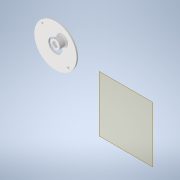
# Autodesk Inventor part: Anglerfish_Lightplate_Tosslink
Saved by Autodesk Inventor 2022 (Build 260153000, 153)
## iProperties
Created: 2022-07-21
Part Number: Anglerfish_Lightplate_Tosslink
Material: Generisch
Document SubType Name: Modeling
Designer: Muriel
Density: 1 g/cm^3
Appearance: Vorgabe
Author: Muriel
Autodesk Inventor part; units mm, degrees
ref_plane "YZ Plane" through (0, 0, 0) normal (1, 0, 0) x (0, 1, 0)
ref_plane "XZ Plane" through (0, 0, 0) normal (0, 1, 0) x (-1, 0, 0)
ref_plane "XY Plane" through (0, 0, 0) normal (0, 0, 1) x (1, 0, 0)
ref_plane "Arbeitsebene1" through (98.0402, -40.0393, 0) normal (0, 0, 1) x (1, 0, 0)
sketch "Skizze1" plane through (98.0402, -40.0393, 0) normal (0, 0, 1) x (1, 0, 0)
  arc A0 (-132.5402, 32.1532) -> (-131.9673, 30.3899) centre (-129.5402, 32.1532) ccw projected
  line L0 (-119.9354, 13.8294) -> (-131.9673, 30.3899) projected
  arc A1 (-119.9354, 13.8294) -> (-118.4354, 12.7395) centre (-117.5083, 15.5927) ccw projected
  line L1 (-98.9673, 6.414) -> (-118.4354, 12.7395) projected
  arc A2 (-98.9673, 6.414) -> (-97.1132, 6.414) centre (-98.0402, 9.2672) ccw projected
  line L2 (-77.6451, 12.7395) -> (-97.1132, 6.414) projected
  arc A3 (-77.6451, 12.7395) -> (-76.1451, 13.8294) centre (-78.5722, 15.5927) ccw projected
  line L3 (-64.1132, 30.3899) -> (-76.1451, 13.8294) projected
  arc A4 (-64.1132, 30.3899) -> (-63.5402, 32.1532) centre (-66.5402, 32.1532) ccw projected
  line L4 (-63.5402, 52.6232) -> (-63.5402, 32.1532) projected
  arc A5 (-63.5402, 52.6232) -> (-64.1132, 54.3865) centre (-66.5402, 52.6232) ccw projected
  line L5 (-76.1451, 70.9471) -> (-64.1132, 54.3865) projected
  arc A6 (-76.1451, 70.9471) -> (-77.6451, 72.0369) centre (-78.5722, 69.1837) ccw projected
  line L6 (-97.1132, 78.3624) -> (-77.6451, 72.0369) projected
  arc A7 (-97.1132, 78.3624) -> (-98.9673, 78.3624) centre (-98.0402, 75.5093) ccw projected
  line L7 (-118.4354, 72.0369) -> (-98.9673, 78.3624) projected
  arc A8 (-118.4354, 72.0369) -> (-119.9354, 70.9471) centre (-117.5083, 69.1837) ccw projected
  line L8 (-131.9673, 54.3865) -> (-119.9354, 70.9471) projected
  arc A9 (-131.9673, 54.3865) -> (-132.5402, 52.6232) centre (-129.5402, 52.6232) ccw projected
  line L9 (-132.5402, 32.1532) -> (-132.5402, 52.6232) projected
  circle A10 centre (-98.0403, 42.3882) radius 10
  arc A11 (-132.5402, 32.1532) -> (-131.9673, 30.3899) centre (-129.5402, 32.1532) ccw projected
  line L10 (-119.9354, 13.8294) -> (-131.9673, 30.3899) projected
  arc A12 (-119.9354, 13.8294) -> (-118.4354, 12.7395) centre (-117.5083, 15.5927) ccw projected
  line L11 (-98.9673, 6.414) -> (-118.4354, 12.7395) projected
  arc A13 (-98.9673, 6.414) -> (-97.1132, 6.414) centre (-98.0402, 9.2672) ccw projected
  line L12 (-77.6451, 12.7395) -> (-97.1132, 6.414) projected
  arc A14 (-77.6451, 12.7395) -> (-76.1451, 13.8294) centre (-78.5722, 15.5927) ccw projected
  line L13 (-64.1132, 30.3899) -> (-76.1451, 13.8294) projected
  arc A15 (-64.1132, 30.3899) -> (-63.5402, 32.1532) centre (-66.5402, 32.1532) ccw projected
  line L14 (-63.5402, 52.6232) -> (-63.5402, 32.1532) projected
  arc A16 (-63.5402, 52.6232) -> (-64.1132, 54.3865) centre (-66.5402, 52.6232) ccw projected
  line L15 (-76.1451, 70.9471) -> (-64.1132, 54.3865) projected
  arc A17 (-76.1451, 70.9471) -> (-77.6451, 72.0369) centre (-78.5722, 69.1837) ccw projected
  line L16 (-97.1132, 78.3624) -> (-77.6451, 72.0369) projected
  arc A18 (-97.1132, 78.3624) -> (-98.9673, 78.3624) centre (-98.0402, 75.5093) ccw projected
  line L17 (-118.4354, 72.0369) -> (-98.9673, 78.3624) projected
  arc A19 (-118.4354, 72.0369) -> (-119.9354, 70.9471) centre (-117.5083, 69.1837) ccw projected
  line L18 (-131.9673, 54.3865) -> (-119.9354, 70.9471) projected
  arc A20 (-131.9673, 54.3865) -> (-132.5402, 52.6232) centre (-129.5402, 52.6232) ccw projected
  line L19 (-132.5402, 32.1532) -> (-132.5402, 52.6232) projected
  circle A21 centre (-88.5403, 53.3903) radius 1.352 projected
  circle A22 centre (-98.0403, 42.3903) radius 3.6574 projected
  circle A23 centre (-98.0403, 42.3903) radius 30
  dimension "d0" = 20
  dimension "d21" = 60
  constraints: 2 centre point, 2 coincident
  measures "d0" diameter of A10
  measures "d21" diameter of A23
extrude "Extrusion1" add sketch "Skizze1" along normal blind 3 contours A21 | A23
sketch "Sketch4" plane through (98.0402, -40.0393, 3) normal (0, 0, 1) x (1, 0, 0)
  circle A0 centre (-88.5403, 53.3903) radius 1.352 projected
  circle A1 centre (-88.5403, 53.3903) radius 3
  point P0 (-98.0402, 40.0393)
  dimension "d20" = 6
  constraints: 1 centre point, 1 coincident
  measures "d20" diameter of A1
extrude "Extrusion4" cut sketch "Sketch4" against normal blind 10 contours A0 | A1
derived "00_toslink_launcher_v3.ipt"
sketch "Sketch6" plane through (98.0402, -40.0393, 3) normal (0, 0, 1) x (1, 0, 0)
  line L0 (-87.0413, 50.1486) -> (-88.0462, 48.8891) projected
  circle A0 centre (-86.7199, 49.7498) radius 0.5 projected
  line L1 (-84.9599, 51.6078) -> (-86.2383, 50.0053) projected
  line L2 (-88.0462, 48.8891) -> (-93.0491, 52.8804) projected
  line L3 (-93.0491, 52.8804) -> (-92.0443, 54.1399) projected
  circle A1 centre (-92.5045, 54.3648) radius 0.5 projected
  line L4 (-92.3357, 54.8697) -> (-91.0884, 56.4331) projected
  line L5 (-92.3357, 54.8697) -> (-92.1057, 54.6862) projected
  line L6 (-91.0884, 56.4331) -> (-90.8585, 56.2497) projected
  circle A2 centre (-98.0403, 42.3882) radius 10 projected
  circle A3 centre (-90.6336, 56.7099) radius 0.5 projected
  line L7 (-89.6815, 57.1016) -> (-90.3122, 56.3111) projected
  line L8 (-89.6815, 57.1016) -> (-88.2761, 57.2597) projected
  line L9 (-88.2761, 57.2597) -> (-84.8366, 54.5157) projected
  line L10 (-84.6362, 53.0766) -> (-84.8366, 54.5157) projected
  line L11 (-85.2357, 52.3251) -> (-84.6362, 53.0766) projected
  circle A4 centre (-84.7754, 52.1003) radius 0.5 projected
  line L12 (-84.9599, 51.6078) -> (-85.1742, 51.7788) projected
  circle A5 centre (-88.5403, 53.3903) radius 4.536
  circle A6 centre (-98.0403, 42.3882) radius 10 projected
  circle A7 centre (-88.5403, 53.3903) radius 6.5
  line L13 (-86.2383, 50.0053) -> (-86.495, 50.2101) projected
  point P0 (-98.0402, 40.0393)
  point P1 (-89.1243, 46.9166)
  point P2 (-94.8598, 51.869)
  point P3 (-86.408, 50.1407)
  point P4 (-87.1107, 50.0617)
  point P5 (-92.114, 54.0526)
  point P6 (-92.1937, 54.7564)
  point P7 (-90.9455, 56.3191)
  point P8 (-90.2428, 56.3981)
  point P9 (-85.1663, 52.4121)
  point P10 (-85.0872, 51.7094)
  point P11 (-89.1243, 46.9166)
  point P12 (-94.8598, 51.869)
  dimension "d17" = 13
  constraints: 4 point on circle, 2 centre point, 1 coincident, 1 tangent, 2 other
  measures "d17" diameter of A7
extrude "Extrusion5" add sketch "Sketch6" along normal blind 10 contours A0 A5 L2 L0 | A0 A5 | L13 L1 L12 A4 L11 L10 L9 L8 L7 A3 L6 L4 L5 A1 A5 A0 | A5 A0 | A2 A7 | A5 A1 L3 | A1 A5 | A1 A5 | A4 | A3 picked at (-82.8002, 54.264)
sketch "Sketch7" plane through (13.2036, 14.4764, 3) normal (-0.6236376, -0.7817136, 0) x (0.7817136, -0.6236376, 0)
  line L0 (0, 7.834) -> (-4.4, 7.834)
  line L1 (-4.4, 7.834) -> (-4.4, 5.6554)
  line L2 (-4.4, 5.6554) -> (0, 5.6554)
  line L3 (0, 5.6554) -> (0, 7.834)
  line L4 (0, 0) -> (0, 10) projected
  line L5 (-4.4, 0) -> (-4.4, 10) projected
  point P0 (-1.2934, -3)
  constraints: 8 end point, 2 parallel, 2 point on line, 1 horizontal, 1 perpendicular
extrude "Extrusion6" cut sketch "Sketch7" against normal blind 1
sketch "Sketch8" plane through (4.9911, 12.8411, 13) normal (0.6236376, 0.7817136, 0) x (0.7817136, -0.6236376, 0)
  line L0 (5.4, 4.3446) -> (1, 4.3446) projected
  line L1 (1, 2.166) -> (5.4, 2.166) projected
  line L2 (5.4, 2.166) -> (5.4, 0) projected
  line L3 (1, 0) -> (5.4, 0) projected
  line L4 (1, 10) -> (1, 4.3446) projected
  line L5 (5.4, 10) -> (1, 10) projected
  line L6 (5.4, 10) -> (5.4, 4.3446) projected
  line L7 (5.4, 4.3446) -> (5.4, 2.166)
  line L8 (1, 2.166) -> (1, 0) projected
  line L9 (1, 4.3446) -> (1, 2.166)
  point P0 (4.1066, 13)
  constraints: 4 end point, 1 collinear, 1 vertical
extrude "Extrusion7" cut sketch "Sketch8" against normal blind 1 contours L7 L1 L9 L0
chamfer "Chamfer1" distance 2 angle 45 1 edges at (13.7479, 18.2708, 3)
sketch "Sketch9" plane through (0, 2.351, 3) normal (0, 0, 1) x (1, 0, 0)
  circle A0 centre (0, -0.0021) radius 25.9979 projected
  arc A1 (9.6814, 2.5019) -> (1.0662, 9.9409) centre (9.4999, 11) ccw projected
  arc A2 (1.0662, 9.9409) -> (9.6814, 2.5019) centre (0, -0.0021) ccw projected
  circle A3 centre (0, 0) radius 30 projected
  circle A4 centre (0, 0) radius 30 projected
  line L0 (0, 0) -> (21.2132, -21.2132)
  line L1 (0, 0) -> (30, 0) construction
  line L2 (21.2132, -21.2132) -> (-21.2132, 21.2132)
  circle A5 centre (-18.3822, 18.3822) radius 1.4
  circle A6 centre (18.3844, -18.3844) radius 1.4
  point P0 (0, -2.351)
  dimension "d29" = 45
  dimension "d30" = 0
  dimension "d31" = 2.8
  dimension "d32" = 2.8
  constraints: 6 end point, 4 point on circle, 2 centre point, 2 point on line, 1 equal length, 1 horizontal
  measures "d29" angle of L0 L1
  measures "d30" distance between parallel lines of L2 L0
  measures "d31" diameter of A5
  measures "d32" diameter of A6
extrude "Extrusion8" cut sketch "Sketch9" against normal through all contours A5 L2 A0 | A0 L2 A5 | A6 L0 A0 | A0 L0 A6 | L2 A5 A0 | A0 A5 L2 | L0 A6 A0 | A0 A6 L0
